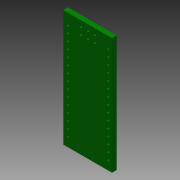
# Autodesk Inventor part: bord
Saved by Autodesk Inventor 2015 (Build 190159000, 159)
## iProperties
Created: 2015-09-08
Part Number: bord
Material: Generic
Document SubType Name: Modeling
Designer: david
Density: 1 g/cm^3
Appearance: Dark Green
Author: david
Autodesk Inventor part; units mm, degrees
ref_plane "YZ Plane" through (0, 0, 0) normal (1, 0, 0) x (0, 1, 0)
ref_plane "XZ Plane" through (0, 0, 0) normal (0, 1, 0) x (-1, 0, 0)
ref_plane "XY Plane" through (0, 0, 0) normal (0, 0, 1) x (1, 0, 0)
sketch "Sketch1" plane through (0, 0, 0) normal (0, 1, 0) x (-1, 0, 0)
  line L0 (9, 21.5) -> (-9, 21.5)
  line L1 (-9, 21.5) -> (-9, -21.5)
  line L2 (-9, -21.5) -> (9, -21.5)
  line L3 (9, -21.5) -> (9, 21.5)
  line L4 (9, 21.5) -> (-9, -21.5) construction
  line L5 (-9, 21.5) -> (9, -21.5) construction
  point P0 (0, 0)
  dimension "d0" = 18
  dimension "d1" = 43
  constraints: 12 end point, 2 midpoint, 2 parallel, 1 horizontal, 1 perpendicular
  measures "d0" distance of L2.end L1.end
  measures "d1" distance of L1.end L0.end
extrude "Extrusion1" add sketch "Sketch1" along normal blind 1.75
sketch "Sketch2" plane through (0, 1.75, 0) normal (0, 1, 0) x (1, 0, 0)
  circle A0 centre (-7.5, -17.5) radius 0.5
  line L0 (-9, -21.5) -> (9, -21.5) projected
  line L1 (-9, 21.5) -> (-9, -21.5) projected
  point P0 (0, 0)
  dimension "d4" = 1
  dimension "d5" = 4
  dimension "d6" = 1.5
  constraints: 1 centre point
  measures "d4" diameter of A0
  measures "d5" distance from line of L0 A0.centre
  measures "d6" distance from line of A0.centre L1
extrude "Extrusion2" cut sketch "Sketch2" against normal blind 1.75
pattern_linear "Rectangular Pattern1" count 15 spacing 2.54 along (0, 0, -1) count 2 spacing 15 along (1, 0, 0) of "Extrusion2"
sketch "Sketch3" plane through (0, 0, 0) normal (0, -1, 0) x (1, 0, 0)
  circle A0 centre (0, 16.96) radius 0.5
  circle A1 centre (0, 19.5) radius 0.5
  circle A2 centre (2.54, 16.96) radius 0.5
  circle A3 centre (2.54, 19.5) radius 0.5
  line L0 (9, -21.5) -> (-9, -21.5) projected
  line L1 (-9, 21.5) -> (9, 21.5) projected
  circle A4 centre (-2.54, 19.5) radius 0.5
  circle A5 centre (-2.54, 16.96) radius 0.5
  point P0 (0, 0)
  dimension "d15" = 1
  dimension "d16" = 1
  dimension "d17" = 2.54
  dimension "d18" = 1
  dimension "d19" = 1
  dimension "d20" = 2.54
  dimension "d23" = 0
  dimension "d24" = 0
  dimension "d25" = 2.54
  dimension "d30" = 0
  dimension "d33" = 2
  dimension "d34" = 1
  dimension "d35" = 1
  dimension "d36" = 1.54
  dimension "d37" = 1.54
  constraints: 6 centre point
  measures "d15" diameter of A0
  measures "d16" diameter of A1
  measures "d17" distance between centres of A0 A1
  measures "d18" diameter of A2
  measures "d19" diameter of A3
  measures "d20" distance between centres of A2 A3
  measures "d23" horizontal distance of A0.centre A1.centre
  measures "d24" horizontal distance of A3.centre A2.centre
  measures "d25" distance of A3.centre A1.centre
  measures "d30" horizontal distance of point (0, 0) A0.centre
  measures "d33" distance from line of L1 A1.centre
  measures "d34" diameter of A4
  measures "d35" diameter of A5
extrude "Extrusion3" cut sketch "Sketch3" against normal blind 10
body "Solid1"
